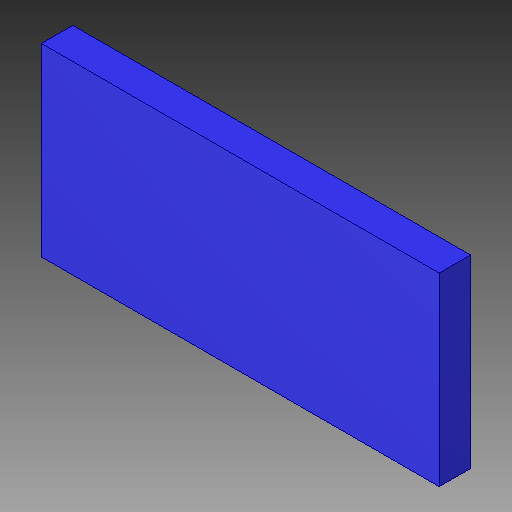
# Autodesk Inventor part: LED_MATRIX
Saved by Autodesk Inventor 2017 (Build 210142000, 142)
## iProperties
Created: 2019-06-13
Part Number: LED_MATRIX
Material: Generic
Document SubType Name: Modeling
Designer: Marc
Density: 1 g/cm^3
Appearance: 6410-05, LED_MATRIX
Author: Marc
Autodesk Inventor part; units mm, degrees
ref_plane "YZ Plane" through (0, 0, 0) normal (1, 0, 0) x (0, 1, 0)
ref_plane "XZ Plane" through (0, 0, 0) normal (0, 1, 0) x (-1, 0, 0)
ref_plane "XY Plane" through (0, 0, 0) normal (0, 0, 1) x (1, 0, 0)
sketch "6410-05, LED_MATRIX_30" plane through (0, 0, 0) normal (0, 0, 1) x (1, 0, 0)
  line L0 (-6.35, 2.9845) -> (6.35, 2.9845)
  line L1 (6.35, 2.9845) -> (6.35, -2.921)
  line L2 (6.35, -2.921) -> (-6.35, -2.921)
  line L3 (-6.35, -2.921) -> (-6.35, 2.9845)
  constraints: 8 end point
extrude "Extrusion1" add sketch "6410-05, LED_MATRIX_30" along normal blind 1
body "Solid1"
